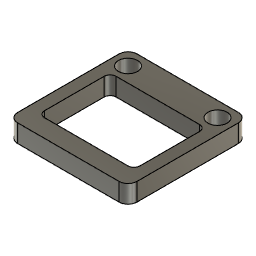
ZSY Standoff (Autodesk Fusion 360 design; units mm, degrees)
Autodesk Fusion 360 part; units mm, degrees
sketch "Sketch1" plane through (0, 0, 0) normal (0, 0, 1) x (1, 0, 0) in component "ZSY Standoff"
  line L0 (0, 0) -> (20, 0)
  line L1 (20, 0) -> (20, 20)
  line L2 (20, 20) -> (0, 20)
  line L3 (0, 20) -> (0, 0)
  line L4 (0, 17.5) -> (20, 17.5) construction
  line L5 (10, 20) -> (10, 0) construction
  circle A0 centre (17.5, 17.5) radius 1.6
  circle A1 centre (2.5, 17.5) radius 1.6
  line L6 (2, 20) -> (2, 0) construction
  line L7 (18, 20) -> (18, 0) construction
  line L8 (0, 3) -> (20, 3) construction
  line L9 (0, 15) -> (20, 15) construction
  line L10 (2, 15) -> (18, 15)
  line L11 (18, 15) -> (18, 3)
  line L12 (18, 3) -> (2, 3)
  line L13 (2, 3) -> (2, 15)
  dimension "d1" = 20
  dimension "d2" = 20
  dimension "d3" = 2.5
  dimension "d4" = 3.2
  dimension "d5" = 3.2
  dimension "d6" = 7.5
  dimension "d7" = 7.5
  dimension "d8" = 2
  dimension "d9" = 2
  dimension "d10" = 3
  dimension "d11" = 5
  constraint horizontal L0
  constraint vertical L1
  constraint horizontal L2
  constraint vertical L3
  constraint coincident L0.start L3.end
  constraint coincident L3 L4.start
  constraint coincident L1 L4.end
  constraint perpendicular L1 L4
  constraint midpoint L2 L5.start
  constraint midpoint L0 L5.end
  constraint coincident L4 A0.centre
  constraint coincident L4 A1.centre
  constraint coincident L2 L6.start
  constraint coincident L0 L6.end
  constraint perpendicular L0 L6
  constraint coincident L2 L7.start
  constraint perpendicular L2 L7
  constraint coincident L3 L8.start
  constraint coincident L1 L8.end
  constraint perpendicular L1 L8
  constraint coincident L3 L9.start
  constraint coincident L1 L9.end
  constraint perpendicular L1 L9
  constraint horizontal L10
  constraint vertical L11
  constraint horizontal L12
  constraint vertical L13
  constraint coincident L8 L11.end
  constraint coincident L7 L11.end
  constraint coincident L9 L10.start
  constraint coincident L6 L10.start
  measures "d1" distance of L0.start L0.end
  measures "d2" distance of L0.start L2.end
  measures "d3" distance of L2 L4
  measures "d4" diameter of A0
  measures "d5" diameter of A1
  measures "d6" distance of L5 A1.centre
  measures "d7" distance of L5 A0.centre
  measures "d8" distance of L3 L6
  measures "d9" distance of L1 L7
  measures "d10" distance of L0 L8
  measures "d11" distance of L2 L9
extrude "Extrude1" add sketch "Sketch1" along normal blind 3 in component "ZSY Standoff"
fillet "Fillet1" radius 1.5 4 edges at (20, 20, 1.5) (0, 20, 1.5) (0, 0, 1.5) (20, 0, 1.5) in component "ZSY Standoff"
fillet "Fillet2" radius 1 4 edges at (2, 15, 1.5) (18, 15, 1.5) (18, 3, 1.5) (2, 3, 1.5) in component "ZSY Standoff"
component "ZSY Standoff" placed x (1, 0, 0) y (0, 1, 0) z (0, 0, 1) at (0, 0, 0)
